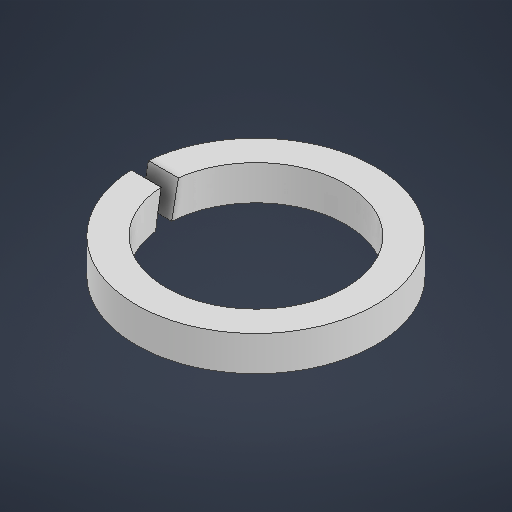
# Autodesk Inventor part: alatet
Saved by Autodesk Inventor 2026.1 (Build 301233020, 233B)
## iProperties
Created: 2025-10-28
Part Number: alatet
Material: Generic
Document SubType Name: Modeling
Designer: User
Density: 1 g/cm^3
Appearance: Default
Author: User
Autodesk Inventor part; units mm, degrees
ref_plane "YZ Plane" through (0, 0, 0) normal (1, 0, 0) x (0, 1, 0)
ref_plane "XZ Plane" through (0, 0, 0) normal (0, 1, 0) x (-1, 0, 0)
ref_plane "XY Plane" through (0, 0, 0) normal (0, 0, 1) x (1, 0, 0)
sketch "Sketch1" plane through (0, 0, 0) normal (0, 1, 0) x (-1, 0, 0)
  circle A0 centre (0, 0) radius 9
  circle A1 centre (0, 0) radius 12
  dimension "d0" = 18
  dimension "d1" = 24
  constraints: 2 centre point, 2 coincident
  measures "d0" diameter of A0
  measures "d1" diameter of A1
extrude "Extrusion1" add sketch "Sketch1" along normal blind 3.5
sketch "Sketch2" plane through (0, 0, 0) normal (1, 0, 0) x (0, 1, 0)
  line L0 (0, 1.1555) -> (3.5, 0.5384)
  line L1 (0, 0) -> (6.1473, 0) construction
  line L2 (0, -0.5267) -> (3.5, -1.1439)
  line L3 (3.5, 0.5384) -> (3.5, -1.1439)
  line L4 (0, -0.5267) -> (0, 1.1555)
  line L5 (3.5, -1.1439) -> (3.5, 0.5384)
  line L6 (3.5, -12) -> (3.5, 12) projected
  line L7 (0, 0) -> (3.554, 0) construction
  constraints: 14 end point, 2 horizontal, 1 collinear
extrude "Extrusion2" cut sketch "Sketch2" against normal blind 300
body "Solid1"
